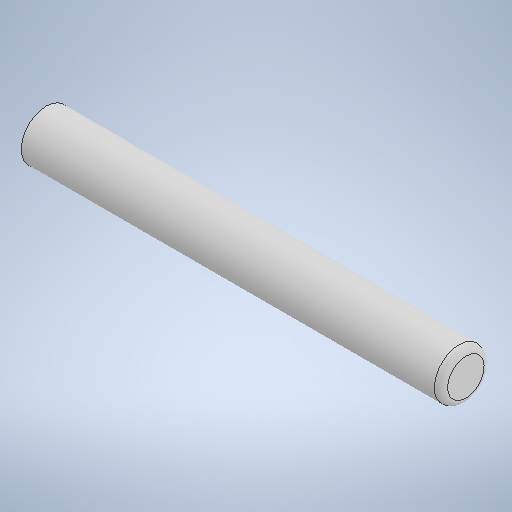
# Autodesk Inventor part: axis
Saved by Autodesk Inventor 2025 (Build 290162000, 162)
## iProperties
Created: 2026-02-12
Part Number: axis
Material: Generic
Document SubType Name: Modeling
Designer: tapen
Density: 1 g/cm^3
Appearance: Default
Author: tapen
Autodesk Inventor part; units mm, degrees
ref_plane "YZ Plane" through (0, 0, 0) normal (1, 0, 0) x (0, 1, 0)
ref_plane "XZ Plane" through (0, 0, 0) normal (0, 1, 0) x (-1, 0, 0)
ref_plane "XY Plane" through (0, 0, 0) normal (0, 0, 1) x (1, 0, 0)
sketch "Sketch1" plane through (0, 0, 0) normal (0, 0, 1) x (1, 0, 0)
  line L0 (0, 7.5) -> (100, 7.5)
  line L1 (100, 7.5) -> (100, 7.5)
  line L2 (126.4895, 0) -> (0, 0)
  line L3 (0, 0) -> (0, 7.5)
  line L4 (100, 7.5) -> (124.4895, 7.5)
  line L5 (126.4895, 5.5) -> (126.4895, 0)
  arc A0 (126.4895, 5.5) -> (124.4895, 7.5) centre (124.4895, 5.5) ccw
  dimension "d0" = 100
  dimension "d2" = 7.5
  dimension "d8" = 2
  constraints: 12 end point, 3 perpendicular, 2 horizontal, 2 point on circle, 2 tangent, 1 centre point, 1 parallel
  measures "d0" distance of L0.start L0.end
  measures "d2" distance of L2.end L0.start
  measures "d8" radius of A0
revolve "Revolution1" add sketch "Sketch1" angle 360 about axis through (126.4895, 0, 0) along (-1, 0, 0)
sketch "Sketch3" plane through (0, 0, 0) normal (-1, 0, 0) x (0, 0, 1)
  circle A0 centre (0, 0) radius 4.07
  dimension "d9" = 8.14
  constraints: 1 centre point, 1 coincident
  measures "d9" diameter of A0
extrude "Extrusion2" cut sketch "Sketch3" against normal blind 3.2
fillet "Fillet1" radius 1 1 edges at (0, 0, -4.07)
body "Solid1"
